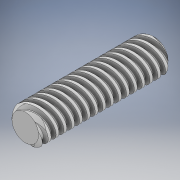
# Autodesk Inventor part: ACME 8mm Lead Screw 2mm-pitch
Saved by Autodesk Inventor 2020.3 (Build 243373000, 373)
## iProperties
Created: 2021-01-08
Part Number: ACME 8mm Lead Screw 2mm-pitch
Material: Generic
Document SubType Name: Modeling
Designer: Johnson Ebenezer R
Density: 1 g/cm^3
Appearance: Default
Author: Johnson Ebenezer R
Autodesk Inventor part; units mm, degrees
ref_plane "YZ Plane" through (0, 0, 0) normal (1, 0, 0) x (0, 1, 0)
ref_plane "XZ Plane" through (0, 0, 0) normal (0, 1, 0) x (-1, 0, 0)
ref_plane "XY Plane" through (0, 0, 0) normal (0, 0, 1) x (1, 0, 0)
sketch "Sketch1" plane through (0, 0, 0) normal (0, 0, 1) x (1, 0, 0)
  circle A0 centre (0, 0) radius 4
  dimension "dia" = 8
  constraints: 1 centre point, 1 coincident
  measures "dia" diameter of A0
extrude "8mm Rod" add sketch "Sketch1" against normal blind 30
chamfer "Chamfer1" distance 0.9071 angle 45 2 edges at (-4, 0, 0) (-4, 0, -30)
sketch "Sketch2" plane through (0, 0, 0) normal (1, 0, 0) x (0, 1, 0)
  line L0 (4, -0.9071) -> (-4, -0.9071) projected
  line L1 (4, 0.6725) -> (3.0929, 0.9071)
  line L2 (3.0929, 0.9071) -> (3.0929, 1.5797)
  line L3 (3.0929, 1.5797) -> (4, 1.8143)
  line L4 (0, 0) -> (0, -30)
  line L5 (3.0929, -30) -> (-3.0929, -30) projected
  line L6 (4, 1.8143) -> (4, 0.6725)
  line L7 (4, 0.6725) -> (4, 0)
  line L8 (-3.0929, 0) -> (3.0929, 0) projected
  dimension "d43" = 1.8143
  dimension "d44" = 0.9071
  dimension "d48" = 29
  constraints: 12 end point, 3 point on line, 3 vertical alignment, 2 equal length, 2 vertical, 1 midpoint
  measures "d43" distance of L3.end L7.end
  measures "d44" distance between parallel lines of L6 L2
  measures "d48" angle of L1 L3
coil "ACME Thread 2mm Pitch" sketch "Sketch2" operation cut axis through (0, 0, 0) along (0, 0, -1) pitch 7.2571 turns 4.383858 hand right
pattern_circular "4 Start" count 4 over 360 about axis through (0, 0, -29.5464) along (0, 0, -1) of "ACME Thread 2mm Pitch"
equation "\"d3\" = 0.5 * p"
equation "\"d43\" = p"
equation "\"d44\" = 0.5 * p"
equation "\"d14\" = 4 * p"
equation "\"p\" = 1.81429"
body "Solid1"
